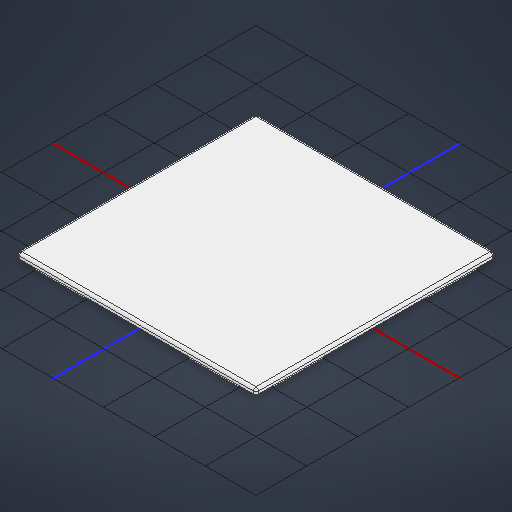
# Autodesk Inventor part: block_main
Saved by Autodesk Inventor 2025.2 (Build 292293000, 293)
## iProperties
Created: 2025-08-04
Part Number: block_main
Material: PC/ABS Plastic
Document SubType Name: Modeling
Designer: sam
Density: 1.1 g/cm^3
Appearance: Smooth - White
Author: sam
Autodesk Inventor part; units mm, degrees
ref_plane "YZ Plane" through (0, 0, 0) normal (1, 0, 0) x (0, 1, 0)
ref_plane "XZ Plane" through (0, 0, 0) normal (0, 1, 0) x (-1, 0, 0)
ref_plane "XY Plane" through (0, 0, 0) normal (0, 0, 1) x (1, 0, 0)
sketch "Sketch4" plane through (0, 0, 0) normal (0, 1, 0) x (-1, 0, 0)
  line L0 (47, 47) -> (-47, 47)
  line L1 (-47, 47) -> (-47, -47)
  line L2 (-47, -47) -> (47, -47)
  line L3 (47, -47) -> (47, 47)
  line L4 (47, 47) -> (-47, -47) construction
  line L5 (-47, 47) -> (47, -47) construction
  point P0 (0, 0)
  dimension "d52" = 94
  dimension "d53" = 94
  constraints: 12 end point, 2 midpoint, 2 parallel, 1 horizontal, 1 perpendicular
  measures "d52" distance of L2.end L1.end
  measures "d53" distance of L1.end L0.end
extrude "Extrusion5" add sketch "Sketch4" along normal blind 2
sketch "Sketch6" plane through (0, 0, 0) normal (0, -1, 0) x (1, 0, 0)
  line L0 (-46.5, -40) -> (-45.5, -40)
  line L1 (-45.5, -40) -> (-45.5, -20)
  line L2 (-45.5, -20) -> (-46.5, -20)
  line L3 (-46.5, -20) -> (-46.5, -40)
  line L4 (-45.5, 20) -> (-46.5, 20)
  line L5 (-46.5, 20) -> (-46.5, 40)
  line L6 (-46.5, 40) -> (-45.5, 40)
  line L7 (-45.5, 40) -> (-45.5, 20)
  line L8 (-40, 46.5) -> (-20, 46.5)
  line L9 (-20, 46.5) -> (-20, 45.5)
  line L10 (-20, 45.5) -> (-40, 45.5)
  line L11 (-40, 45.5) -> (-40, 46.5)
  line L12 (40, 46.5) -> (20, 46.5)
  line L13 (20, 46.5) -> (20, 45.5)
  line L14 (20, 45.5) -> (40, 45.5)
  line L15 (40, 45.5) -> (40, 46.5)
  line L16 (45.5, 40) -> (46.5, 40)
  line L17 (46.5, 40) -> (46.5, 20)
  line L18 (46.5, 20) -> (45.5, 20)
  line L19 (45.5, 20) -> (45.5, 40)
  line L20 (45.5, -40) -> (46.5, -40)
  line L21 (46.5, -40) -> (46.5, -20)
  line L22 (46.5, -20) -> (45.5, -20)
  line L23 (45.5, -20) -> (45.5, -40)
  line L24 (40, -45.5) -> (20, -45.5)
  line L25 (20, -45.5) -> (20, -46.5)
  line L26 (20, -46.5) -> (40, -46.5)
  line L27 (40, -46.5) -> (40, -45.5)
  line L28 (-40, -45.5) -> (-20, -45.5)
  line L29 (-20, -45.5) -> (-20, -46.5)
  line L30 (-20, -46.5) -> (-40, -46.5)
  line L31 (-40, -46.5) -> (-40, -45.5)
  line L32 (-47, 47) -> (-47, -47)
  line L33 (47, 47) -> (-47, 47)
  line L34 (47, -47) -> (47, 47)
  line L35 (-47, -47) -> (47, -47)
  point P0 (0, 0)
  point P1 (-46, 40)
  point P2 (-46, 20)
  point P3 (46, 40)
  point P4 (46, -40)
  point P5 (-40, -46)
  point P6 (-46, -40)
  dimension "d123" = 1
  dimension "d124" = 20
  dimension "d119" = 1
  dimension "d118" = 20
  dimension "d116" = 20
  dimension "d117" = 1
  dimension "d112" = 20
  dimension "d113" = 1
  dimension "d108" = 1
  dimension "d109" = 20
  dimension "d104" = 1
  dimension "d105" = 20
  dimension "d101" = 20
  dimension "d102" = 1
  dimension "d97" = 20
  dimension "d98" = 1
  dimension "d114" = 7
  dimension "d115" = 0.5
  dimension "d111" = 0.5
  dimension "d110" = 7
  dimension "d107" = 7
  dimension "d106" = 0.5
  dimension "d103" = 0.5
  dimension "d95" = 7
  dimension "d99" = 7
  dimension "d100" = 0.5
  dimension "d96" = 0.5
  dimension "d94" = 7
  dimension "d93" = 7
  dimension "d122" = 0.5
  dimension "d120" = 7
  dimension "d121" = 0.5
  constraints: 72 end point, 14 parallel, 7 horizontal, 7 perpendicular, 6 midpoint
  measures "d123" distance of L2.end L1.end
  measures "d124" distance of L1.end L0.end
  measures "d119" distance between parallel lines of L7 L5
  measures "d118" distance of point (-46, 40) point (-46, 20)
  measures "d116" distance of L9.end L10.end
  measures "d117" distance of L8.end L9.end
  measures "d112" distance of L14.end L13.end
  measures "d113" distance of L13.end L12.end
  measures "d108" distance of L17.end L18.end
  measures "d109" distance of L16.end L17.end
  measures "d104" distance of L22.end L21.end
  measures "d105" distance of L21.end L20.end
  measures "d101" distance of L26.end L25.end
  measures "d102" distance of L25.end L24.end
  measures "d97" distance of L29.end L30.end
  measures "d98" distance of L28.end L29.end
  measures "d114" distance between parallel lines of L32 L11
  measures "d115" distance between parallel lines of L33 L8
  measures "d111" distance between parallel lines of L33 L12
  measures "d110" distance between parallel lines of L34 L15
  measures "d107" distance between parallel lines of L33 L16
  measures "d106" distance between parallel lines of L34 L17
  measures "d103" distance between parallel lines of L34 L21
  measures "d95" distance from line of L35 point (46, -40)
  measures "d99" distance between parallel lines of L34 L27
  measures "d100" distance between parallel lines of L35 L26
  measures "d96" distance between parallel lines of L35 L30
  measures "d94" distance from line of L32 point (-40, -46)
  measures "d93" distance from line of L35 point (-46, -40)
  measures "d122" distance between parallel lines of L32 L3
  measures "d120" distance between parallel lines of L33 L6
  measures "d121" distance between parallel lines of L32 L5
extrude "Extrusion7" add sketch "Sketch6" along normal blind 1 contours L3 L2 L1 L0 | L4 L5 L6 L7 | L8 L9 L10 L11 | L15 L14 L13 L12 | L16 L17 L18 L19 | L23 L22 L21 L20 | L27 L26 L25 L24 | L28 L29 L30 L31
fillet "Fillet9" radius 1 1 edges at (47, 1, -47)
fillet "Fillet10" radius 1 1 edges at (-47, 1, -47)
fillet "Fillet11" radius 1 1 edges at (-47, 1, 47)
fillet "Fillet12" radius 1 1 edges at (47, 1, 47)
fillet "Fillet13" radius 1 8 edges at (-46.7071, 2, -46.7071) (-47, 2, 0) (-46.7071, 2, 46.7071) (0, 2, 47) (46.7071, 2, 46.7071) (47, 2, 0) (46.7071, 2, -46.7071) (0, 2, -47)
body "Solid1"
